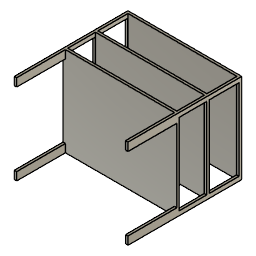
bathroom mini shelf v1 (Autodesk Fusion 360 design; units mm, degrees)
Autodesk Fusion 360 part; units mm, degrees
sketch "Sketch1" plane through (0, 0, 0) normal (0, 0, 1) x (1, 0, 0)
  line L0 (0, 0) -> (140, 0)
  line L1 (140, 0) -> (140, 140)
  line L2 (140, 140) -> (0, 140)
  line L3 (0, 140) -> (0, 0)
  dimension "d1" = 140
  dimension "d2" = 140
  constraint horizontal L0
  constraint vertical L1
  constraint horizontal L2
  constraint vertical L3
  constraint coincident L0.start L3.end
  measures "d1" distance of L0.start L0.end
  measures "d2" distance of L0.start L2.end
extrude "Extrude1" add sketch "Sketch1" along normal blind 110
sketch "Sketch2" plane through (0, 0, 110) normal (0, 0, 1) x (-1, 0, 0)
  line L0 (0, -140) -> (0, 0)
  line L1 (0, 0) -> (-140, 0)
  line L2 (-140, 0) -> (-140, -140)
  line L3 (-140, -140) -> (0, -140)
  line L4 (0, -140) -> (-3, -140)
  line L5 (-3, -140) -> (-3, -137)
  line L6 (-3, -137) -> (0, -137)
  line L7 (0, -137) -> (0, -140)
  line L8 (-70, -140) -> (-70, 0)
  line L9 (0, -100) -> (-140, -100)
  line L10 (0, -60) -> (-140, -60)
  line L11 (-137, -137) -> (-140, -137)
  line L12 (-137, -140) -> (-137, -137)
  line L13 (-3, -63) -> (0, -63)
  line L14 (-3, -60) -> (-3, -63)
  line L15 (-137, -60) -> (-137, -63)
  line L16 (-137, -63) -> (-140, -63)
  line L17 (0, -100) -> (-3, -100)
  line L18 (-3, -100) -> (-3, -97)
  line L19 (-3, -97) -> (0, -97)
  line L20 (0, -97) -> (0, -100)
  line L21 (0, -100) -> (-140, -100)
  line L22 (-140, -100) -> (-140, -97)
  line L23 (-140, -97) -> (0, -97)
  line L24 (0, -97) -> (0, -100)
  line L25 (-140, -60) -> (0, -60)
  line L26 (0, -60) -> (0, -63)
  line L27 (0, -63) -> (-140, -63)
  line L28 (-140, -63) -> (-140, -60)
  line L29 (-140, -140) -> (0, -140)
  line L30 (0, -140) -> (0, -137)
  line L31 (0, -137) -> (-140, -137)
  line L32 (-140, -137) -> (-140, -140)
  line L33 (0, -140) -> (-3, -140)
  line L34 (-3, -140) -> (-3, 0)
  line L35 (-3, 0) -> (0, 0)
  line L36 (0, 0) -> (0, -140)
  line L37 (-140, -140) -> (-137, -140)
  line L38 (-137, -140) -> (-137, 0)
  line L39 (-137, 0) -> (-140, 0)
  line L40 (-140, 0) -> (-140, -140)
  dimension "d5" = 3
  dimension "d6" = 3
  dimension "d7" = 3
  dimension "d8" = 3
  constraint horizontal L4
  constraint vertical L5
  constraint horizontal L6
  constraint vertical L7
  constraint coincident L0.start L3.end
  constraint midpoint L3 L8.start
  constraint midpoint L1 L8.end
  constraint coincident L0 L9.start
  constraint coincident L2 L9.end
  constraint perpendicular L2 L9
  constraint coincident L0 L10.start
  constraint coincident L2 L10.end
  constraint perpendicular L2 L10
  constraint symmetric L4.end L8 L12.start
  constraint symmetric L5.end L8 L11.start
  constraint symmetric L6.end L8 L11.end
  constraint symmetric L4.end L9 L14.start
  constraint symmetric L5.end L9 L13.start
  constraint symmetric L6.end L9 L13.end
  constraint symmetric L9 L11.start L15.end
  constraint symmetric L9 L11.end L16.end
  constraint symmetric L9 L12.start L15.start
  constraint horizontal L17
  constraint vertical L18
  constraint horizontal L19
  constraint vertical L20
  constraint horizontal L21
  constraint vertical L22
  constraint horizontal L23
  constraint vertical L24
  constraint coincident L2 L22.end
  constraint horizontal L25
  constraint vertical L26
  constraint horizontal L27
  constraint vertical L28
  constraint horizontal L29
  constraint vertical L30
  constraint horizontal L31
  constraint vertical L32
  constraint coincident L2.end L3.start
  constraint horizontal L33
  constraint vertical L34
  constraint horizontal L35
  constraint vertical L36
  constraint coincident L1 L34.end
  constraint horizontal L37
  constraint vertical L38
  constraint horizontal L39
  constraint vertical L40
  constraint coincident L1 L38.end
  measures "d5" distance of L0.start L4.end
  measures "d6" distance of L0.start L6.end
  measures "d7" distance of L9.start L17.end
  measures "d8" distance of L9.start L19.end
extrude "Extrude2" cut sketch "Sketch2" against normal blind 110 contours L8 L9 L21 L31 L34 | L8 L9 L21 L31 L38 | L8 L23 L27 L34 | L8 L23 L27 L38 | L1 L8 L10 L25 L34 | L1 L8 L10 L25 L38
sketch "Sketch3" plane through (140, 0, 0) normal (1, 0, 0) x (0, 1, 0)
  line L0 (0, 0) -> (140, 0)
  line L1 (140, 0) -> (140, 110)
  line L2 (140, 110) -> (0, 110)
  line L3 (0, 110) -> (0, 0)
  line L4 (0, 110) -> (10, 110)
  line L5 (10, 110) -> (10, 100)
  line L6 (10, 100) -> (0, 100)
  line L7 (0, 100) -> (0, 110)
  line L8 (0, 0) -> (10, 0)
  line L9 (10, 0) -> (10, 10)
  line L10 (10, 10) -> (0, 10)
  line L11 (0, 10) -> (0, 0)
  line L12 (60, 110) -> (50, 110)
  line L13 (50, 110) -> (50, 100)
  line L14 (50, 100) -> (60, 100)
  line L15 (60, 100) -> (60, 110)
  line L16 (60, 0) -> (50, 0)
  line L17 (50, 0) -> (50, 10)
  line L18 (50, 10) -> (60, 10)
  line L19 (60, 10) -> (60, 0)
  line L20 (50, 10) -> (10, 10)
  line L21 (10, 10) -> (10, 100)
  line L22 (10, 100) -> (50, 100)
  line L23 (50, 100) -> (50, 10)
  line L24 (60, 100) -> (60, 10)
  constraint horizontal L4
  constraint vertical L5
  constraint horizontal L6
  constraint vertical L7
  constraint coincident L2.end L3.start
  constraint horizontal L8
  constraint vertical L9
  constraint horizontal L10
  constraint vertical L11
  constraint coincident L0.start L3.end
  constraint horizontal L12
  constraint vertical L13
  constraint horizontal L14
  constraint vertical L15
  constraint coincident L2 L12.start
  constraint horizontal L16
  constraint vertical L17
  constraint horizontal L18
  constraint vertical L19
  constraint coincident L0 L16.start
  constraint horizontal L20
  constraint vertical L21
  constraint horizontal L22
  constraint vertical L23
  constraint perpendicular L18 L24
extrude "Extrude3" cut sketch "Sketch3" against normal blind 140 contours L3 L6 L10 L21 | L20 L21 L22 L23 | L14 L18 L23 L24
sketch "Sketch5" plane through (0, 0, 0) normal (-1, 0, 0) x (0, -1, 0)
  line L0 (0, 10) -> (-60, 10)
  line L1 (-60, 10) -> (-60, 100)
  line L2 (-60, 100) -> (0, 100)
  line L3 (0, 100) -> (0, 110)
  line L4 (0, 110) -> (-140, 110)
  line L5 (-140, 110) -> (-140, 0)
  line L6 (-140, 0) -> (0, 0)
  line L7 (0, 0) -> (0, 10)
  line L8 (-136.5713, 0) -> (-100, 0)
  line L9 (-100, 0) -> (-100, 110)
  line L10 (-100, 110) -> (-136.5713, 110)
  line L11 (-136.5713, 110) -> (-136.5713, 0)
  line L12 (-136.5713, 5.3179) -> (-100, 5.3179)
  line L13 (-100, 5.3179) -> (-100, 105)
  line L14 (-100, 105) -> (-136.5713, 105)
  line L15 (-136.5713, 105) -> (-136.5713, 5.3179)
  line L16 (-96.7286, 0) -> (-63.0271, 0)
  line L17 (-63.0271, 0) -> (-63.0271, 110)
  line L18 (-63.0271, 110) -> (-96.7286, 110)
  line L19 (-96.7286, 110) -> (-96.7286, 0)
  line L20 (-96.7286, 5.3179) -> (-63.0271, 5.3179)
  line L21 (-63.0271, 5.3179) -> (-63.0271, 104.8767)
  line L22 (-63.0271, 104.8767) -> (-96.7286, 104.8767)
  line L23 (-96.7286, 104.8767) -> (-96.7286, 5.3179)
  constraint horizontal L8
  constraint vertical L9
  constraint horizontal L10
  constraint vertical L11
  constraint coincident L4 L9.end
  constraint coincident L6 L8.start
  constraint horizontal L12
  constraint vertical L13
  constraint horizontal L14
  constraint vertical L15
  constraint coincident L9 L13.end
  constraint coincident L11 L12.start
  constraint horizontal L16
  constraint vertical L17
  constraint horizontal L18
  constraint vertical L19
  constraint coincident L4 L17.end
  constraint coincident L6 L16.start
  constraint horizontal L20
  constraint vertical L21
  constraint horizontal L22
  constraint vertical L23
  constraint coincident L17 L21.end
  constraint coincident L19 L20.start
extrude "Extrude4" cut sketch "Sketch5" against normal blind 140 contours L17 L19 L20 L21 L22 L23 | L9 L11 L12 L13 L14 L15
